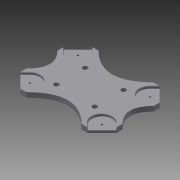
# Autodesk Inventor part: plaque
Saved by Autodesk Inventor 2015 (Build 190159000, 159)
## iProperties
Created: 2015-02-17
Part Number: plaque
Material: Generic
Document SubType Name: Modeling
Designer: Piotr
Density: 1 g/cm^3
Appearance: Default
Mass: 255.612 g
Surface Area: 638.979 cm^2
Volume: 255.612 cm^3
Author: Piotr
Autodesk Inventor part; units mm, degrees
ref_plane "YZ Plane" through (0, 0, 0) normal (1, 0, 0) x (0, 1, 0)
ref_plane "XZ Plane" through (0, 0, 0) normal (0, 1, 0) x (-1, 0, 0)
ref_plane "XY Plane" through (0, 0, 0) normal (0, 0, 1) x (1, 0, 0)
sketch "Sketch2" plane through (0, 0, 0) normal (0, 0, 1) x (1, 0, 0)
  line L0 (-100, 75) -> (100, 75)
  line L1 (100, 75) -> (100, -75)
  line L2 (100, -75) -> (-100, -75)
  line L3 (-100, -75) -> (-100, 75)
  line L4 (157.6027, 0) -> (-257.5856, 0) construction
  line L5 (0, 44.2956) -> (0, -158.1506) construction
  point P0 (0, 0)
  dimension "d0" = 200
  dimension "d1" = 150
  constraints: 12 end point, 2 horizontal, 2 parallel, 2 point on line, 1 perpendicular, 1 vertical, 2 other
  measures "d0" distance of L0.start L0.end
  measures "d1" distance of L0.end L1.end
extrude "Extrusion1" add sketch "Sketch2" along normal blind 10
sketch "Sketch3" plane through (0, 0, 0) normal (0, 0, -1) x (-1, 0, 0)
  line L0 (-100, 45) -> (-70, 75)
  line L1 (-100, 75) -> (100, 75) projected
  line L2 (-100, 75) -> (-100, -75) projected
  line L3 (100, 75) -> (-100, 75) projected
  point P0 (0, 0)
  dimension "d4" = 45
  dimension "d5" = 30
  constraints: 3 point on line, 2 end point
  measures "d4" angle of L1 L0
  measures "d5" horizontal distance of L0.start L0.end
split body "Split1" sketch "Sketch3" result one side removed curves L0 removed pieces at (90, 65, 0.5)
mirror "Mirror1" about plane through (0, 0, 0) normal (0, 1, 0) of "Split1"
mirror "Mirror2" about plane through (0, 0, 0) normal (1, 0, 0) of "Split1", "Mirror1"
sketch "Sketch4" plane through (0, 0, 10) normal (0, 0, 1) x (1, 0, 0)
  line L0 (100, 45) -> (90, 35)
  line L1 (100, 45) -> (70, 75) projected
  line L2 (90, 35) -> (25.0224, 99.9776) construction
  arc A0 (60, 65) -> (90, 35) centre (75, 50) ccw
  line L3 (70, 75) -> (60, 65)
  line L4 (70, 75) -> (100, 45)
  point P0 (0, 0)
  dimension "d17" = 10
  constraints: 8 end point, 2 parallel, 2 perpendicular, 2 point on circle, 2 point on line, 1 centre point
  measures "d17" horizontal distance of L0.start L0.end
extrude "Extrusion2" cut sketch "Sketch4" against normal blind 5
sketch "Sketch5" plane through (0, 0, 5) normal (0, 0, 1) x (1, 0, 0)
  circle A0 centre (75, 50) radius 2
  arc A1 (60, 65) -> (90, 35) centre (75, 50) ccw projected
  point P0 (0, 0)
  dimension "d9" = 4
  constraints: 1 centre point, 1 concentric
  measures "d9" diameter of A0
hole "Hole1" at (75, 50, 5) direction (0, 0, -1) diameter 4 end through all
chamfer "Chamfer3" distance 1 angle 45 3 edges at (65, 70, 10) (60, 35, 10) (95, 40, 10)
mirror "Mirror3" about plane through (0, 0, 0) normal (0, 1, 0) of "Extrusion2", "Hole1", "Chamfer3"
mirror "Mirror4" about plane through (0, 0, 0) normal (1, 0, 0) of "Extrusion2", "Hole1", "Mirror3", "Chamfer3"
sketch "Sketch6" plane through (0, 0, 10) normal (0, 0, 1) x (1, 0, 0)
  circle A0 centre (40, 30) radius 5
  point P0 (0, 0)
  dimension "d18" = 30
  dimension "d19" = 40
  dimension "d20" = 10
  constraints: 1 centre point
  measures "d18" vertical distance of point (0, 0) A0.centre
  measures "d19" horizontal distance of point (0, 0) A0.centre
  measures "d20" diameter of A0
extrude "Extrusion3" cut sketch "Sketch6" against normal blind 8.5
hole "Hole2" at (40, 30, 1.5) direction (0, 0, -1) diameter 7 end through all
mirror "Mirror5" about plane through (0, 0, 0) normal (0, 1, 0) of "Hole2", "Extrusion3"
mirror "Mirror6" about plane through (0, 0, 0) normal (1, 0, 0) of "Hole2", "Extrusion3", "Mirror5"
sketch "Sketch7" plane through (0, 0, 10) normal (0, 0, 1) x (1, 0, 0)
  line L0 (-100, 43.5858) -> (-90.7071, 34.2929) construction
  line L1 (-90.7071, -34.2929) -> (-100, -43.5858) construction
  line L2 (-100, 43.5858) -> (-100, -43.5858) projected
  line L3 (-100, 32.2721) -> (-67.7279, 0) construction
  line L4 (-67.7279, 0) -> (-100, -32.2721) construction
  spline S0 degree 2 poles (-100, 32.2721) (-67.7279, 0) (-100, -32.2721) knots 1 1 1 2 2 2
  line L5 (-58.7752, 0) -> (-112.5381, 0) construction
  point P0 (0, 0)
  dimension "d41" = 8
  constraints: 4 point on line, 2 end point, 2 parallel, 1 horizontal, 1 symmetric about line, 3 other
  measures "d41" distance between parallel lines of L0 L3
extrude "Extrusion4" cut sketch "Sketch7" against normal blind 10
mirror "Mirror7" about plane through (0, 0, 0) normal (1, 0, 0) of "Extrusion4"
sketch "Sketch9" plane through (0, 0, 10) normal (0, 0, 1) x (1, 0, 0)
  line L0 (-68.5858, -75) -> (68.5858, -75) construction
  line L1 (-57.2721, -75) -> (0, -17.7279) construction
  line L2 (0, -17.7279) -> (57.2721, -75) construction
  spline S0 degree 2 poles (-57.2721, -75) (0, -17.7279) (57.2721, -75) knots 1 1 1 2 2 2
  line L3 (-68.5858, -75) -> (-59.2929, -65.7071) construction
  line L4 (59.2929, -65.7071) -> (68.5858, -75) construction
  line L5 (-57.2721, -75) -> (57.2721, -75)
  line L6 (70, -75) -> (-70, -75) projected
  point P0 (0, 0)
  dimension "d44" = 8
  dimension "d45" = 8
  constraints: 2 end point, 2 parallel, 2 point on line, 1 collinear, 3 other
  measures "d44" distance between parallel lines of L4 L2
  measures "d45" distance between parallel lines of L1 L3
extrude "Extrusion5" cut sketch "Sketch9" against normal blind 10
mirror "Mirror8" about plane through (0, 0, 0) normal (0, 1, 0) of "Extrusion5"
body "Solid1"
